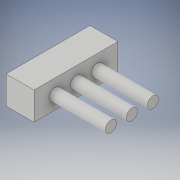
# Autodesk Inventor part: Part2
Saved by Autodesk Inventor 2019 (Build 230136000, 136)
## iProperties
Created: 2018-12-13
Part Number: Part2
Material: Generic
Document SubType Name: Modeling
Designer: User
Density: 1 g/cm^3
Appearance: Default
Author: User
Autodesk Inventor part; units mm, degrees
ref_plane "YZ Plane" through (0, 0, 0) normal (1, 0, 0) x (0, 1, 0)
ref_plane "XZ Plane" through (0, 0, 0) normal (0, 1, 0) x (-1, 0, 0)
ref_plane "XY Plane" through (0, 0, 0) normal (0, 0, 1) x (1, 0, 0)
sketch "Sketch1" plane through (0, 0, 0) normal (1, 0, 0) x (0, 1, 0)
  line L0 (0, 0) -> (25.4, 0)
  line L1 (25.4, 0) -> (25.4, 76.2)
  line L2 (25.4, 76.2) -> (0, 76.2)
  line L3 (0, 76.2) -> (0, 0)
  dimension "d2" = 25.4
  dimension "d3" = 76.2
  constraints: 8 end point, 2 parallel, 1 horizontal, 1 perpendicular
  measures "d2" distance of L1.end L2.end
  measures "d3" distance of L0.end L1.end
extrude "Extrusion1" add sketch "Sketch1" along normal blind 25.4
sketch "Sketch2" plane through (25.4, 0, 0) normal (1, 0, 0) x (0, 0, -1)
  circle A0 centre (-717.1181, 162.0804) radius 50.8
  circle A1 centre (-57.15, 12.7) radius 5.08
  circle A2 centre (-38.1, 12.7) radius 5.08
  circle A3 centre (-19.05, 12.7) radius 5.08
  line L0 (0, 25.4) -> (-76.2, 25.4) projected
  line L1 (-76.2, 0) -> (0, 0) projected
  line L2 (-76.2, 25.4) -> (-76.2, 0) projected
  line L3 (0, 0) -> (0, 25.4) projected
  dimension "d6" = 101.6
  dimension "d15" = 10.16
  dimension "d16" = 10.16
  dimension "d17" = 10.16
  dimension "d18" = 25.4
  dimension "d19" = 12.7
  dimension "d21" = 76.2
  dimension "d22" = 38.1
  dimension "d23" = 19.05
  dimension "d24" = 25.4
  dimension "d26" = 19.05
  dimension "d27" = 12.7
  constraints: 4 centre point, 1 horizontal alignment
  measures "d6" diameter of A0
  measures "d15" diameter of A1
  measures "d16" diameter of A2
  measures "d17" diameter of A3
  measures "d18" distance between parallel lines of L1 L0
  measures "d19" distance from line of L0 A1.centre
  measures "d21" distance of L0.start L0.end
  measures "d22" distance from line of L3 A2.centre
  measures "d23" distance from line of L3 A3.centre
  measures "d24" distance of L0.end L1.start
  measures "d26" distance of A2.centre A1.centre
  measures "d27" distance from line of L0 A2.centre
extrude "Extrusion2" add sketch "Sketch2" along normal blind 50.8 contours A1 | A2 | A3
equation "\"d16\" = d15"
equation "\"d17\" = d15"
equation "\"d19\" = 0.5 * d18"
equation "\"d22\" = 0.5 * d21"
equation "\"d23\" = 0.5 * d22"
equation "\"d26\" = d23"
equation "\"d27\" = d19"
body "Solid1"
